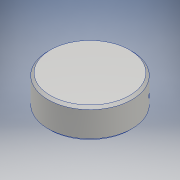
# Autodesk Inventor part: dummy_disc
Saved by Autodesk Inventor 2017 (Build 210142000, 142)
## iProperties
Created: 2017-09-28
Part Number: dummy_disc
Material: Aluminum 6061
Document SubType Name: Modeling
Designer: Thoma
Density: 2.7 g/cm^3
Appearance: Aluminum - Flat
Author: Thoma
Autodesk Inventor part; units mm, degrees
sketch "Sketch1" plane through (0, 0, 0) normal (0, 0, 1) x (1, 0, 0)
  circle A0 centre (0, 0) radius 35
  dimension "d0" = 70
  constraints: 1 centre point, 1 coincident
  measures "d0" diameter of A0
extrude "Extrusion1" add sketch "Sketch1" along normal blind 25
chamfer "Chamfer1" distance 2 angle 45 2 edges at (-35, 0, 25) (-35, 0, 0)
sketch "Sketch2" plane through (0, 0, 25) normal (0, 0, 1) x (1, 0, 0)
  line L0 (0, 0) -> (0, 35) construction
  circle A0 centre (0, 0) radius 35 construction
  line L1 (0, 0) -> (35, 0) construction
  line L2 (0, 0) -> (26.8116, 22.4976) construction
  line L3 (0, 0) -> (35, 0) construction
  line L4 (0, 0) -> (17.5, 30.3109) construction
  line L5 (0, 0) -> (35, 0) construction
  line L6 (0, 0) -> (-26.8116, 22.4976) construction
  line L7 (0, 0) -> (-17.5, 30.3109) construction
  dimension "d6" = 40
  dimension "d7" = 60
  dimension "d48" = 60
  constraints: 16 end point, 4 point on circle, 2 equal length, 2 horizontal, 2 symmetric about line, 1 perpendicular
  measures "d6" angle of L3 L2
  measures "d7" angle of L5 L4
  measures "d48" angle of L3 L7
ref_plane "Work Plane1" through (26.8116, 22.4976, 25) normal (0.766, 0.6428, 0) x (-0.6428, 0.766, 0)
ref_plane "Work Plane2" through (17.5, 30.3109, 25) normal (0.5, 0.866, 0) x (-0.866, 0.5, 0)
ref_plane "Work Plane3" through (-17.5, 30.3109, 25) normal (-0.5, 0.866, 0) x (-0.866, -0.5, 0)
ref_plane "Work Plane4" through (-26.8116, 22.4976, 25) normal (-0.766, 0.6428, 0) x (-0.6428, -0.766, 0)
sketch "Sketch3" plane through (26.8116, 22.4976, 25) normal (0.766, 0.6428, 0) x (-0.6428, 0.766, 0)
  line L0 (-33, 0) -> (33, 0) projected
  point P0 (0, -25)
  point P1 (0, -14.5)
  dimension "d8" = 14.5
  measures "d8" distance from line of point (0, -14.5) L0
sketch "Sketch4" plane through (17.5, 30.3109, 25) normal (0.5, 0.866, 0) x (-0.866, 0.5, 0)
  line L0 (-33, 0) -> (33, 0) projected
  point P0 (0, -25)
  point P1 (0, -14.5)
  dimension "d9" = 14.5
  measures "d9" distance from line of L0 point (0, -14.5)
sketch "Sketch5" plane through (-17.5, 30.3109, 25) normal (-0.5, 0.866, 0) x (-0.866, -0.5, 0)
  line L0 (-33, 0) -> (33, 0) projected
  point P0 (0, -25)
  point P1 (0, -14.5)
  dimension "d10" = 14.5
  measures "d10" distance from line of L0 point (0, -14.5)
sketch "Sketch6" plane through (-26.8116, 22.4976, 25) normal (-0.766, 0.6428, 0) x (-0.6428, -0.766, 0)
  line L0 (-33, 0) -> (33, 0) projected
  point P0 (0, -25)
  point P1 (0, -14.5)
  dimension "d11" = 14.5
  measures "d11" distance from line of L0 point (0, -14.5)
hole "Hole1" at (-26.8116, 22.4976, 10.5) direction (0.766, -0.6428, 0) diameter 3 depth 8 tip angle 118
hole "Hole2" at (-17.5, 30.3109, 10.5) direction (0.5, -0.866, 0) diameter 3 depth 8 tip angle 118
hole "Hole3" at (17.5, 30.3109, 10.5) direction (-0.5, -0.866, 0) diameter 3 depth 8 tip angle 118
hole "Hole4" at (26.8116, 22.4976, 10.5) direction (-0.766, -0.6428, 0) diameter 3 depth 8 tip angle 118
thread "Thread1" size "M3x0.5" class "6H" standard "ANSI Metric M Profile" full length
thread "Thread2" size "M3x0.5" class "6H" standard "ANSI Metric M Profile" full length
thread "Thread3" size "M3x0.5" class "6H" standard "ANSI Metric M Profile" full length
thread "Thread4" size "M3x0.5" class "6H" standard "ANSI Metric M Profile" full length
body "Solid1"
